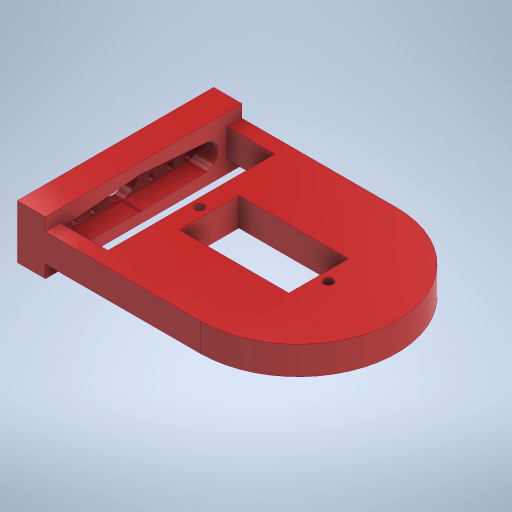
# Autodesk Inventor part: unions2s3pt
Saved by Autodesk Inventor 2024.3 (Build 283343000, 343)
## iProperties
Created: 2025-08-10
Part Number: unions2s3pt
Material: Generic
Document SubType Name: Modeling
Designer: jscme
Density: 1 g/cm^3
Appearance: Default
Author: jscme
Autodesk Inventor part; units mm, degrees
ref_plane "YZ Plane" through (0, 0, 0) normal (1, 0, 0) x (0, 1, 0)
ref_plane "XZ Plane" through (0, 0, 0) normal (0, 1, 0) x (-1, 0, 0)
ref_plane "XY Plane" through (0, 0, 0) normal (0, 0, 1) x (1, 0, 0)
sketch "Sketch1" plane through (0, 0, 0) normal (0, 1, 0) x (-1, 0, 0)
  arc A0 (-33.02, 20.955) -> (-33.02, -20.955) centre (-33.02, 0) ccw
  line L0 (0, 20.955) -> (-33.02, 20.955)
  line L1 (-33.02, -20.955) -> (0, -20.955)
  line L2 (-13.979695, 6.35) -> (-37.347695, 6.35)
  line L3 (-37.347695, 6.35) -> (-37.347695, -6.35)
  line L4 (-37.347695, -6.35) -> (-13.979695, -6.35)
  line L5 (-13.979695, -6.35) -> (-13.979695, 6.35)
  circle A1 centre (-39.430495, 0) radius 1.016
  circle A2 centre (-11.896895, 0) radius 1.016
  line L6 (0, 20.955) -> (0, -20.955)
  point P0 (0, 0)
  point P1 (0, 0)
  point P2 (-37.347695, 0)
  dimension "d1" = 41.91
  dimension "d3" = 12.7
  dimension "d4" = 23.368
  dimension "d5" = 2.032
  dimension "d6" = 2.032
  dimension "d7" = 2.0828
  dimension "d8" = 2.0828
  dimension "d9" = 6.4105
  dimension "d87" = 33.02
  dimension "d88" = 33.02
  constraints: 14 end point, 4 horizontal alignment, 3 centre point, 2 coincident, 2 horizontal, 2 midpoint, 2 parallel, 2 point on circle, 2 tangent, 1 perpendicular
  measures "d1" diameter of A0
  measures "d3" distance of L4.end L2.start
  measures "d4" distance of L3.end L4.end
  measures "d5" diameter of A2
  measures "d6" diameter of A1
  measures "d7" distance from line of A2.centre L5
  measures "d8" distance from line of L3 A1.centre
  measures "d9" distance of A0.centre A1.centre
  measures "d87" distance of L1.start L1.end
  measures "d88" distance of L0.start L0.end
extrude "Extrusion1" add sketch "Sketch1" along normal blind 6
sketch "Sketch4" plane through (0, 0, -20.955) normal (-1, 0, 0) x (0, 0, 1)
  line L0 (41.91, 8.715) -> (0, 8.715)
  line L1 (0, 8.715) -> (0, -2.715)
  line L2 (0, -2.715) -> (41.91, -2.715)
  line L3 (41.91, -2.715) -> (41.91, 8.715)
  line L4 (0, 0) -> (41.91, 0) projected
  line L5 (41.91, 0) -> (41.91, 6) projected
  point P0 (20.955, 0)
  point P1 (20.955, -2.715)
  point P2 (20.955, 0)
  point P3 (41.91, 3)
  point P4 (41.91, 3)
  dimension "d43" = 41.91
  dimension "d44" = 11.43
  constraints: 8 end point, 4 midpoint, 2 parallel, 1 coincident, 1 horizontal, 1 perpendicular, 1 vertical alignment
  measures "d43" distance of L1.end L2.end
  measures "d44" distance between parallel lines of L2 L0
extrude "Extrusion4" add sketch "Sketch4" along normal blind 6
sketch "Sketch8" plane through (0, 6, 0) normal (0, 1, 0) x (1, 0, 0)
  line L0 (0, -17.78) -> (10.16, -17.78)
  line L1 (10.16, -17.78) -> (10.16, 17.78)
  line L2 (10.16, 17.78) -> (0, 17.78)
  line L3 (0, 17.78) -> (0, -17.78)
  line L4 (0, -20.955) -> (0, 20.955) projected
  point P0 (0, 0)
  point P1 (0, 0)
  point P2 (0, 0)
  point P3 (0, 0)
  point P4 (0, 0)
  point P5 (0, 0)
  dimension "d74" = 10.16
  dimension "d75" = 35.56
  constraints: 8 end point, 5 midpoint, 2 coincident, 2 parallel, 1 horizontal, 1 perpendicular
  measures "d74" distance of L1.end L2.end
  measures "d75" distance of L0.end L1.end
extrude "Extrusion10" cut sketch "Sketch8" against normal blind 16.999991
sketch "Sketch12" plane through (-6, 0, -20.955) normal (-1, 0, 0) x (0, 0, 1)
  line L0 (0, 8.715) -> (0, -2.715)
  line L1 (41.91, -2.715) -> (41.91, 8.715)
  arc A0 (35.512447, 0.300645) -> (35.512447, 5.699355) centre (35.37098, 3) ccw
  line L2 (21.59, -0.429) -> (35.512447, 0.300645)
  line L3 (21.59, 6.429) -> (35.512447, 5.699355)
  circle A1 centre (21.59, 3) radius 3.429
  line L4 (21.59, -0.429) -> (6.703499, 0.351168)
  line L5 (21.59, 6.429) -> (6.703499, 5.648832)
  arc A2 (6.703499, 5.648832) -> (6.703499, 0.351168) centre (6.842318, 3) ccw
  circle A3 centre (15.187051, 3) radius 0.75
  circle A4 centre (11.187051, 3) radius 0.75
  circle A5 centre (7.187051, 3) radius 0.75
  line L6 (21.59, 10.756719) -> (21.59, -4.756719)
  circle A6 centre (27.992949, 3) radius 0.75
  circle A7 centre (31.992949, 3) radius 0.75
  circle A8 centre (35.992949, 3) radius 0.75
  point P0 (34.925, 2)
  point P1 (34.925, 2)
  point P2 (34.925, 2)
  point P3 (14.859, -1.175)
  point P4 (14.859, 5.175)
  point P5 (34.925, 2)
  point P6 (41.91, 3)
  point P7 (38.07404, 3)
  point P8 (41.91, 3)
  point P9 (21.231572, 6.410216)
  point P10 (21.231572, -0.410216)
  point P11 (21.948428, -0.410216)
  point P12 (21.948428, 6.410216)
  point P13 (6.205131, 2.479358)
  point P14 (9.863981, 3)
  point P15 (5.48634, 2.396716)
  point P16 (4.189851, 3)
  point P17 (0, 3)
  point P18 (0, 3)
  point P19 (41.91, 3)
  dimension "d143" = 6
  dimension "d144" = 6.858
  dimension "d145" = 6
  dimension "d146" = 13.78098
  dimension "d147" = 20.32
  dimension "d156" = 1.5
  dimension "d157" = 1.5
  dimension "d158" = 1.5
  dimension "d159" = 4
  dimension "d160" = 4
  dimension "d161" = 2.9972
  dimension "d162" = 17.40015
  constraints: 10 end point, 9 centre point, 8 horizontal alignment, 8 point on circle, 3 midpoint, 3 symmetric about line, 3 tangent, 2 vertical alignment, 1 coincident, 1 equal length, 1 vertical, 7 other
  measures "d143" angle of L4 L5
  measures "d144" diameter of A1
  measures "d145" angle of L3 L2
  measures "d146" distance of A0.centre A1.centre
  measures "d156" diameter of A5
  measures "d157" diameter of A4
  measures "d158" diameter of A3
  measures "d159" distance of A5.centre A4.centre
  measures "d160" distance of A4.centre A3.centre
  measures "d161" distance of point (4.19, 3) A5.centre
  measures "d162" distance of A1.centre point (4.19, 3)
sketch "Sketch12 outline for Extrusion13" plane through (-6, 0, -20.955) normal (-1, 0, 0) x (0, 0, 1)
  line L0 (21.59, 6.429) -> (21.231572, 6.410216)
  line L1 (21.948428, 6.410216) -> (21.59, 6.429)
  arc A0 (21.948428, -0.410216) -> (21.948428, 6.410216) centre (21.59, 3) ccw
  line L2 (21.59, -0.429) -> (21.948428, -0.410216)
  line L3 (21.231572, -0.410216) -> (21.59, -0.429)
  arc A1 (21.231572, 6.410216) -> (21.231572, -0.410216) centre (21.59, 3) ccw
extrude "Extrusion13" cut sketch "Sketch12 outline for Extrusion13" against normal blind 8.762492
sketch "Sketch17" plane through (0, 0, -20.955) normal (1, 0, 0) x (0, 0, -1)
  arc A0 (-7.753278, -0.143381) -> (-7.582189, 5.248432) centre (-7.80902, 2.557009) ccw
  line L0 (-21.59, -0.429) -> (-7.753278, -0.143381)
  line L1 (-21.59, 6.429) -> (-7.582189, 5.248432)
  circle A1 centre (-21.59, 3) radius 3.429
  line L2 (-21.59, -0.429) -> (-36.606269, -0.19851)
  line L3 (-21.59, 6.429) -> (-36.548101, 5.0886)
  arc A2 (-36.548101, 5.0886) -> (-36.606269, -0.19851) centre (-36.310948, 2.442116) ccw
  arc A3 (-21.231572, -0.410216) -> (-21.231572, 6.410216) centre (-21.59, 3) ccw
  circle A4 centre (-27.970676, 2.471347) radius 0.75
  circle A5 centre (-31.970676, 2.471347) radius 0.75
  circle A6 centre (-35.970676, 2.471347) radius 0.75
  line L4 (-21.59, 6.429) -> (-21.59, -0.429)
  circle A7 centre (-15.209324, 2.471347) radius 0.75
  circle A8 centre (-11.209324, 2.471347) radius 0.75
  circle A9 centre (-7.209324, 2.471347) radius 0.75
  point P0 (-20.955, 0)
  point P1 (-16.352581, -1.161112)
  point P2 (-16.352581, 5.188888)
  point P3 (-5.109414, 2.471347)
  point P4 (-21.695241, -0.427385)
  point P5 (-22.199652, 6.374369)
  point P6 (-21.016089, 6.380631)
  point P7 (-21.448497, -0.426079)
  point P8 (-30.453399, 2.232188)
  point P9 (-26.794548, 2.471347)
  point P10 (-31.172189, 2.149546)
  point P11 (-38.967876, 2.471347)
  dimension "d150" = 6
  dimension "d151" = 6.858
  dimension "d152" = 6
  dimension "d153" = 13.78098
  dimension "d163" = 1.5
  dimension "d164" = 1.5
  dimension "d165" = 1.5
  dimension "d166" = 4
  dimension "d167" = 4
  dimension "d168" = 2.9972
  constraints: 10 end point, 9 centre point, 8 point on circle, 5 horizontal alignment, 3 symmetric about line, 3 tangent, 2 vertical alignment, 1 concentric, 1 equal length, 3 other
  measures "d150" angle of L2 L3
  measures "d151" diameter of A1
  measures "d152" angle of L1 L0
  measures "d153" horizontal distance of A0.centre A1.centre
  measures "d163" diameter of A6
  measures "d164" diameter of A5
  measures "d165" diameter of A4
  measures "d166" distance of A6.centre A5.centre
  measures "d167" distance of A5.centre A4.centre
  measures "d168" distance of point (-38.968, 2.471) A6.centre
sketch "Sketch17 outline for Extrusion17" plane through (0, 0, -20.955) normal (1, 0, 0) x (0, 0, -1)
  arc A0 (-36.548101, 5.0886) -> (-36.606269, -0.19851) centre (-36.310948, 2.442116) ccw
  line L0 (-22.199652, 6.374369) -> (-36.548101, 5.0886)
  arc A1 (-21.695241, -0.427385) -> (-22.199652, 6.374369) centre (-21.59, 3) cw
  line L1 (-36.606269, -0.19851) -> (-21.695241, -0.427385)
  arc A2 (-7.753278, -0.143381) -> (-7.582189, 5.248432) centre (-7.80902, 2.557009) ccw
  line L2 (-21.448497, -0.426079) -> (-7.753278, -0.143381)
  arc A3 (-21.016089, 6.380631) -> (-21.448497, -0.426079) centre (-21.59, 3) cw
  line L3 (-7.582189, 5.248432) -> (-21.016089, 6.380631)
extrude "Extrusion17" cut sketch "Sketch17 outline for Extrusion17" against normal blind 4
sketch "Sketch19" plane through (-4, 0, -20.955) normal (1, 0, 0) x (0, 0, -1)
  circle A0 centre (-27.7378, 0.757495) radius 0.75
  circle A1 centre (-31.7378, 0.757495) radius 0.75
  circle A2 centre (-35.7378, 0.757495) radius 0.75
  line L0 (-38.735, 6) -> (-38.735, 3.530276)
  line L1 (-21.564652, 3.265138) -> (-21.564652, -1.203525)
  circle A3 centre (-15.391504, 0.757495) radius 0.75
  circle A4 centre (-11.391504, 0.757495) radius 0.75
  circle A5 centre (-7.391504, 0.757495) radius 0.75
  point P0 (-20.955, 0)
  point P1 (-32.395372, 0.835812)
  point P2 (-31.71002, 0.757495)
  point P3 (-38.735, 1.75317)
  point P4 (-38.735, 4.765138)
  dimension "d169" = 1.5
  dimension "d170" = 1.5
  dimension "d171" = 1.5
  dimension "d172" = 4
  dimension "d173" = 4
  dimension "d174" = 2.9972
  constraints: 6 centre point, 3 horizontal alignment, 3 symmetric about line, 2 end point, 1 midpoint, 1 vertical, 1 vertical alignment, 3 other
  measures "d169" diameter of A2
  measures "d170" diameter of A1
  measures "d171" diameter of A0
  measures "d172" distance of A2.centre A1.centre
  measures "d173" distance of A1.centre A0.centre
  measures "d174" horizontal distance of point (-38.735, 4.765) A2.centre
extrude "Extrusion18" cut sketch "Sketch19" against normal blind 25.4
body "Solid1"
